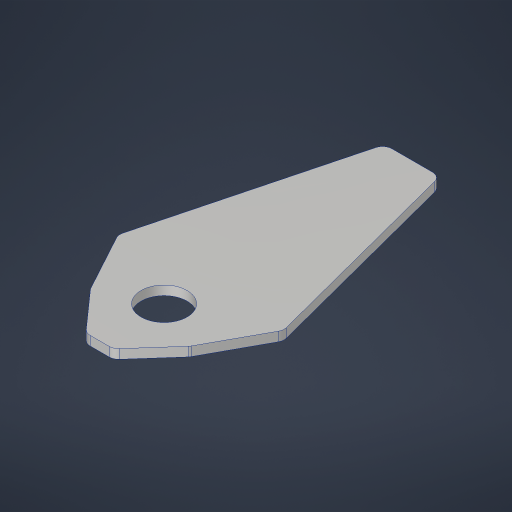
# Autodesk Inventor part: CL4-003
Saved by Autodesk Inventor 2023.4 (Build 274418000, 418)
## iProperties
Created: 2025-02-03
Part Number: CL4-003
Material: Aluminum 6061
Document SubType Name: Modeling
Designer: brand
Density: 2.7 g/cm^3
Appearance: Aluminum - Flat
Author: brand
Autodesk Inventor part; units mm, degrees
ref_plane "YZ Plane" through (0, 0, 0) normal (1, 0, 0) x (0, 1, 0)
ref_plane "XZ Plane" through (0, 0, 0) normal (0, 1, 0) x (-1, 0, 0)
ref_plane "XY Plane" through (0, 0, 0) normal (0, 0, 1) x (1, 0, 0)
sketch "Sketch1" plane through (0, 0, 0) normal (0, 1, 0) x (-1, 0, 0)
  line L0 (19.05, -215.9) -> (-19.05, -215.9)
  line L1 (-19.05, -215.9) -> (-57.15, -69.85)
  line L2 (19.05, -215.9) -> (57.15, -69.85)
  line L3 (57.15, -69.85) -> (19.05, 0)
  line L4 (19.05, 0) -> (-19.05, 0)
  line L5 (-19.05, 0) -> (-57.15, -69.85)
  line L6 (57.15, -69.85) -> (-57.15, -69.85) construction
  line L7 (-12.7, -50.8) -> (12.7, -50.8) construction
  line L8 (12.7, -50.8) -> (12.7, 0) construction
  line L9 (12.7, 0) -> (-12.7, 0) construction
  line L10 (-12.7, 0) -> (-12.7, -50.8) construction
  point P0 (0, 0)
  point P1 (0, -215.9)
  point P2 (0, -69.85)
  point P3 (0, 0)
  dimension "d0" = 25.4
  dimension "d1" = 50.8
  dimension "d2" = 6.35
  dimension "d3" = 114.3
  dimension "d4" = 215.9
  dimension "d5" = 19.05
  dimension "d6" = 38.1
  constraints: 22 end point, 4 horizontal, 4 midpoint, 2 coincident, 2 parallel, 2 vertical alignment, 1 horizontal alignment, 1 perpendicular
  measures "d0" distance of L7.start L7.end
  measures "d1" distance of L7.end L8.end
  measures "d2" distance of L4.end L9.end
  measures "d3" distance of L2.end L1.end
  measures "d4" distance from line of L8.end L0
  measures "d5" distance between parallel lines of L7 L6
  measures "d6" distance of L0.start L0.end
extrude "Extrusion1" add sketch "Sketch1" along normal mid plane 6.35
fillet "Fillet1" radius 6.604 4 edges at (57.15, 0, -69.85) (19.05, 0, -215.9) (-19.05, 0, -215.9) (-57.15, 0, -69.85)
fillet "Fillet2" [suppressed]
sketch "Sketch2" plane through (0, 3.175, 0) normal (0, 1, 0) x (1, 0, 0)
  arc A0 (20.3379, 210.963) -> (13.9478, 215.9) centre (13.9478, 209.296) ccw construction
  line L0 (20.3379, 210.963) -> (56.4895, 72.3821) construction
  arc A1 (55.8969, 67.5527) -> (56.4895, 72.3821) centre (50.0993, 70.7151) ccw construction
  line L1 (55.8969, 67.5527) -> (19.05, 0) construction
  line L2 (-19.05, 0) -> (-55.8969, 67.5527) construction
  arc A2 (-56.4895, 72.3821) -> (-55.8969, 67.5527) centre (-50.0993, 70.7151) ccw construction
  line L3 (-56.4895, 72.3821) -> (-20.3379, 210.963) construction
  arc A3 (-13.9478, 215.9) -> (-20.3379, 210.963) centre (-13.9478, 209.296) ccw construction
  line L4 (-13.9478, 215.9) -> (13.9478, 215.9) construction
  line L5 (13.9478, 215.9) -> (-13.9478, 215.9) construction
  line L6 (19.05, 0) -> (-19.05, 0) projected
  point P0 (0, 44.45)
  point P1 (0, 215.9)
  point P2 (0, 215.9)
  constraints: 2 midpoint, 2 vertical alignment
hole "Hole1" at (0, 3.175, -44.45) direction (0, -1, 0) diameter 31.75 end through all
chamfer "Chamfer1" distance 9.525 distance2 31.75 2 edges at (19.05, 0, 0) (-19.05, 0, 0) measured on face at (-18.55, 0, 0) measured on face at (18.55, 0, 0)
fillet "Fillet3" radius 6.604 4 edges at (9.525, 0, 0) (34.2536, 0, -27.8732) (-9.525, 0, 0) (-34.2536, 0, -27.8732)
equation "\"d23\" = d9"
equation "\"d9\" = 6.604"
body "Solid1"
